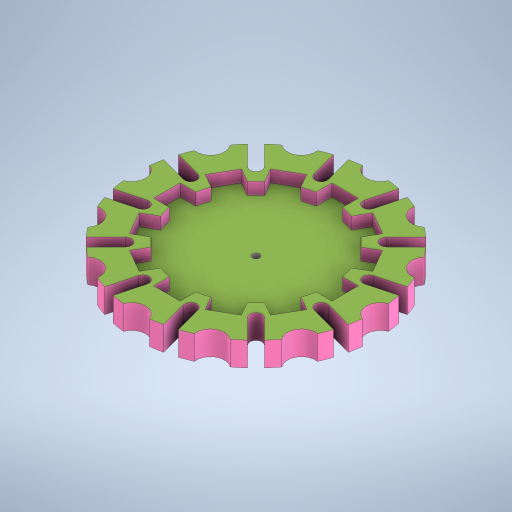
# Autodesk Inventor part: Geneva Gear 12
Saved by Autodesk Inventor 2023 (Build 270158000, 158)
## iProperties
Created: 2022-10-22
Part Number: Geneva Gear 12
Material: Generic
Document SubType Name: Modeling
Designer: annah
Density: 1 g/cm^3
Appearance: Default
Author: annah
Autodesk Inventor part; units mm, degrees
ref_plane "YZ Plane" through (0, 0, 0) normal (1, 0, 0) x (0, 1, 0)
ref_plane "XZ Plane" through (0, 0, 0) normal (0, 1, 0) x (-1, 0, 0)
ref_plane "XY Plane" through (0, 0, 0) normal (0, 0, 1) x (1, 0, 0)
sketch "Sketch1" plane through (0, 0, 0) normal (0, 1, 0) x (-1, 0, 0)
  line L0 (19.1342, -46.194) -> (0, -54.1231)
  line L1 (0, -54.1231) -> (0, 0)
  line L2 (0, 0) -> (19.1342, -46.194)
  circle A0 centre (0, 0) radius 50
  line L3 (17.2491, -28.6141) -> (23.8838, -44.6316)
  circle A1 centre (0, -54.1231) radius 20.712
  arc A2 (17.5355, -29.3054) -> (8.1665, -32.7812) centre (12.7859, -30.8678) ccw
  line L4 (14.5151, -48.1081) -> (8.1665, -32.7812)
  line L5 (19.1342, -41.194) -> (0, -41.194)
  circle A3 centre (0, -54.1231) radius 12.9291
  arc A4 (-11.6961, -48.6128) -> (11.6961, -48.6128) centre (0, 0) ccw
  arc A5 (-11.6961, -48.6128) -> (11.6961, -48.6128) centre (0, -54.1231) ccw
  circle A6 centre (0, -54.1231) radius 32.5
  arc A7 (19.1342, -41.194) -> (16.6765, -41.8397) centre (19.1342, -46.194) ccw
  arc A8 (14.4249, -47.874) -> (23.5974, -43.9403) centre (19.1342, -46.194) ccw
  line L6 (32.4302, -8.0362) -> (48.4477, -14.6709)
  arc A9 (33.1215, -8.3226) -> (28.9544, -17.4053) centre (30.8678, -12.7859) ccw
  line L7 (44.2813, -23.7539) -> (28.9544, -17.4053)
  arc A10 (44.052, -23.6521) -> (47.7564, -14.3846) centre (46.194, -19.1342) ccw
  circle A11 centre (38.2708, -38.2708) radius 12.9291
  line L8 (28.6141, 17.2491) -> (44.6316, 23.8838)
  arc A12 (29.3054, 17.5355) -> (32.7812, 8.1665) centre (30.8678, 12.7859) ccw
  line L9 (48.1081, 14.5151) -> (32.7812, 8.1665)
  arc A13 (47.874, 14.4249) -> (43.9403, 23.5974) centre (46.194, 19.1342) ccw
  circle A14 centre (54.1231, 0) radius 12.9291
  line L10 (8.0362, 32.4302) -> (14.6709, 48.4477)
  arc A15 (8.3226, 33.1215) -> (17.4053, 28.9544) centre (12.7859, 30.8678) ccw
  line L11 (23.7539, 44.2813) -> (17.4053, 28.9544)
  arc A16 (23.6521, 44.052) -> (14.3846, 47.7564) centre (19.1342, 46.194) ccw
  circle A17 centre (38.2708, 38.2708) radius 12.9291
  line L12 (-17.2491, 28.6141) -> (-23.8838, 44.6316)
  arc A18 (-17.5355, 29.3054) -> (-8.1665, 32.7812) centre (-12.7859, 30.8678) ccw
  line L13 (-14.5151, 48.1081) -> (-8.1665, 32.7812)
  arc A19 (-14.4249, 47.874) -> (-23.5974, 43.9403) centre (-19.1342, 46.194) ccw
  circle A20 centre (0, 54.1231) radius 12.9291
  line L14 (-32.4302, 8.0362) -> (-48.4477, 14.6709)
  arc A21 (-33.1215, 8.3226) -> (-28.9544, 17.4053) centre (-30.8678, 12.7859) ccw
  line L15 (-44.2813, 23.7539) -> (-28.9544, 17.4053)
  arc A22 (-44.052, 23.6521) -> (-47.7564, 14.3846) centre (-46.194, 19.1342) ccw
  circle A23 centre (-38.2708, 38.2708) radius 12.9291
  line L16 (-28.6141, -17.2491) -> (-44.6316, -23.8838)
  arc A24 (-29.3054, -17.5355) -> (-32.7812, -8.1665) centre (-30.8678, -12.7859) ccw
  line L17 (-48.1081, -14.5151) -> (-32.7812, -8.1665)
  arc A25 (-47.874, -14.4249) -> (-43.9403, -23.5974) centre (-46.194, -19.1342) ccw
  circle A26 centre (-54.1231, 0) radius 12.9291
  line L18 (-8.0362, -32.4302) -> (-14.6709, -48.4477)
  arc A27 (-8.3226, -33.1215) -> (-17.4053, -28.9544) centre (-12.7859, -30.8678) ccw
  line L19 (-23.7539, -44.2813) -> (-17.4053, -28.9544)
  arc A28 (-23.6521, -44.052) -> (-14.3846, -47.7564) centre (-19.1342, -46.194) ccw
  circle A29 centre (-38.2708, -38.2708) radius 12.9291
  circle A30 centre (0, 0) radius 3.5
  circle A31 centre (0, -54.1231) radius 3.5
  arc A32 (-7.5, -54.1231) -> (7.5, -54.1231) centre (0, -54.1231) ccw
  arc A33 (7.5, 0) -> (-7.5, 0) centre (0, 0) ccw
  line L20 (7.5, 0) -> (7.5, -54.1231)
  line L21 (-7.5, 0) -> (-7.5, -54.1231)
  circle A34 centre (0, -33.4111) radius 5
  point P0 (8.1662, -32.7805)
  point P1 (23.5974, -43.9403)
  point P2 (28.9537, -17.405)
  point P3 (29.1285, -29.1285)
  point P4 (26.1041, -42.6448)
  point P5 (42.6448, -26.1041)
  point P6 (32.7805, 8.1662)
  point P7 (41.194, 0)
  point P8 (48.6128, -11.6961)
  point P9 (48.6128, 11.6961)
  point P10 (17.405, 28.9537)
  point P11 (29.1285, 29.1285)
  point P12 (42.6448, 26.1041)
  point P13 (26.1041, 42.6448)
  point P14 (-8.1662, 32.7805)
  point P15 (0, 41.194)
  point P16 (11.6961, 48.6128)
  point P17 (-11.6961, 48.6128)
  point P18 (-28.9537, 17.405)
  point P19 (-29.1285, 29.1285)
  point P20 (-26.1041, 42.6448)
  point P21 (-42.6448, 26.1041)
  point P22 (-32.7805, -8.1662)
  point P23 (-41.194, 0)
  point P24 (-48.6128, 11.6961)
  point P25 (-48.6128, -11.6961)
  point P26 (-17.405, -28.9537)
  point P27 (-29.1285, -29.1285)
  point P28 (-42.6448, -26.1041)
  point P29 (-26.1041, -42.6448)
  point P30 (23.6521, -44.052)
  point P31 (26.1041, -42.6448)
  point P32 (42.6448, -26.1041)
  point P33 (44.049, -23.6577)
  point P34 (47.874, -14.4249)
  point P35 (48.6128, -11.6961)
  point P36 (48.6128, 11.6961)
  point P37 (47.8758, 14.4189)
  point P38 (44.052, 23.6521)
  point P39 (42.6448, 26.1041)
  point P40 (26.1041, 42.6448)
  point P41 (23.6577, 44.049)
  point P42 (14.4249, 47.874)
  point P43 (11.6961, 48.6128)
  point P44 (-11.6961, 48.6128)
  point P45 (-14.4189, 47.8758)
  point P46 (-23.6521, 44.052)
  point P47 (-26.1041, 42.6448)
  point P48 (-42.6448, 26.1041)
  point P49 (-44.049, 23.6577)
  point P50 (-47.874, 14.4249)
  point P51 (-48.6128, 11.6961)
  point P52 (-48.6128, -11.6961)
  point P53 (-47.8758, -14.4189)
  point P54 (-44.052, -23.6521)
  point P55 (-42.6448, -26.1041)
  point P56 (-26.1041, -42.6448)
  point P57 (-23.6577, -44.049)
  point P58 (-14.4249, -47.874)
  point P59 (14.4189, -47.8758)
  dimension "d2" = 100
  dimension "d3" = 22.5
  dimension "d4" = 20.712
  dimension "d5" = 50
  dimension "d6" = 54.1231
  dimension "d7" = 10
  dimension "d8" = 25.8582
  dimension "d9" = 65
  dimension "d10" = 360
  dimension "d11" = 7
  dimension "d12" = 7
  dimension "d13" = 15
  dimension "d14" = 15
  dimension "d15" = 10
  constraints: 113 point on circle, 44 end point, 35 centre point, 28 point on line, 9 coincident, 3 tangent, 2 vertical, 1 concentric, 1 parallel, 1 perpendicular, 161 other
  measures "d2" diameter of A0
  measures "d3" angle of L2 L1
  measures "d4" distance of L0.start L0.end
  measures "d5" distance of L1.end L0.start
  measures "d6" distance of L0.end L1.end
  measures "d7" diameter of A2
  measures "d8" diameter of A3
  measures "d9" diameter of A6
  measures "d11" diameter of A30
  measures "d12" diameter of A31
  measures "d13" diameter of A32
  measures "d14" diameter of A33
  measures "d15" diameter of A34
sketch "Sketch2" plane through (0, 0, 0) normal (0, 1, 0) x (-1, 0, 0)
  circle A0 centre (0, 0) radius 100
  line L0 (0, 0) -> (18.5658, -69.2885)
  line L1 (0, 0) -> (0, -103.5276)
  arc A1 (24.6448, -72.6673) -> (14.9907, -75.2542) centre (0, 0) ccw
  circle A2 centre (25.8819, -96.5926) radius 5
  arc A3 (24.729, -72.9816) -> (15.0747, -75.5678) centre (19.8599, -74.1181) ccw
  line L2 (30.6777, -95.1782) -> (24.6448, -72.6673)
  line L3 (21.0523, -97.8867) -> (14.9907, -75.2542)
  circle A4 centre (0, -103.5276) radius 11.6229
  line L4 (21.0523, -97.8867) -> (25.8819, -96.5926)
  arc A5 (-25.8819, -96.5926) -> (26.7197, -101.5219) centre (0, -103.5276) ccw
  circle A6 centre (0, -103.5276) radius 40
  arc A7 (57.9067, -50.8394) -> (50.8389, -57.9063) centre (54.2582, -54.2582) ccw
  line L5 (67.1751, -74.2462) -> (50.6094, -57.6767)
  line L6 (74.1567, -67.0879) -> (57.6767, -50.6094)
  circle A8 centre (70.7107, -70.7107) radius 5
  circle A9 centre (51.7638, -89.6575) radius 11.6229
  arc A10 (75.5684, -15.0748) -> (72.9809, -24.7289) centre (74.1181, -19.8599) ccw
  line L7 (95.2985, -30.7115) -> (72.6673, -24.6448)
  line L8 (97.7655, -21.0214) -> (75.2542, -14.9907)
  circle A11 centre (96.5926, -25.8819) radius 5
  circle A12 centre (89.6575, -51.7638) radius 11.6229
  arc A13 (72.9816, 24.729) -> (75.5678, 15.0747) centre (74.1181, 19.8599) ccw
  line L9 (97.8867, 21.0523) -> (75.2542, 14.9907)
  line L10 (95.1782, 30.6777) -> (72.6673, 24.6448)
  circle A14 centre (96.5926, 25.8819) radius 5
  circle A15 centre (103.5276, 0) radius 11.6229
  arc A16 (50.8394, 57.9067) -> (57.9063, 50.8389) centre (54.2582, 54.2582) ccw
  line L11 (74.2462, 67.1751) -> (57.6767, 50.6094)
  line L12 (67.0879, 74.1567) -> (50.6094, 57.6767)
  circle A17 centre (70.7107, 70.7107) radius 5
  circle A18 centre (89.6575, 51.7638) radius 11.6229
  arc A19 (15.0748, 75.5684) -> (24.7289, 72.9809) centre (19.8599, 74.1181) ccw
  line L13 (30.7115, 95.2985) -> (24.6448, 72.6673)
  line L14 (21.0214, 97.7655) -> (14.9907, 75.2542)
  circle A20 centre (25.8819, 96.5926) radius 5
  circle A21 centre (51.7638, 89.6575) radius 11.6229
  arc A22 (-24.729, 72.9816) -> (-15.0747, 75.5678) centre (-19.8599, 74.1181) ccw
  line L15 (-21.0523, 97.8867) -> (-14.9907, 75.2542)
  line L16 (-30.6777, 95.1782) -> (-24.6448, 72.6673)
  circle A23 centre (-25.8819, 96.5926) radius 5
  circle A24 centre (0, 103.5276) radius 11.6229
  arc A25 (-57.9067, 50.8394) -> (-50.8389, 57.9063) centre (-54.2582, 54.2582) ccw
  line L17 (-67.1751, 74.2462) -> (-50.6094, 57.6767)
  line L18 (-74.1567, 67.0879) -> (-57.6767, 50.6094)
  circle A26 centre (-70.7107, 70.7107) radius 5
  circle A27 centre (-51.7638, 89.6575) radius 11.6229
  arc A28 (-75.5684, 15.0748) -> (-72.9809, 24.7289) centre (-74.1181, 19.8599) ccw
  line L19 (-95.2985, 30.7115) -> (-72.6673, 24.6448)
  line L20 (-97.7655, 21.0214) -> (-75.2542, 14.9907)
  circle A29 centre (-96.5926, 25.8819) radius 5
  circle A30 centre (-89.6575, 51.7638) radius 11.6229
  arc A31 (-72.9816, -24.729) -> (-75.5678, -15.0747) centre (-74.1181, -19.8599) ccw
  line L21 (-97.8867, -21.0523) -> (-75.2542, -14.9907)
  line L22 (-95.1782, -30.6777) -> (-72.6673, -24.6448)
  circle A32 centre (-96.5926, -25.8819) radius 5
  circle A33 centre (-103.5276, 0) radius 11.6229
  arc A34 (-50.8394, -57.9067) -> (-57.9063, -50.8389) centre (-54.2582, -54.2582) ccw
  line L23 (-74.2462, -67.1751) -> (-57.6767, -50.6094)
  line L24 (-67.0879, -74.1567) -> (-50.6094, -57.6767)
  circle A35 centre (-70.7107, -70.7107) radius 5
  circle A36 centre (-89.6575, -51.7638) radius 11.6229
  arc A37 (-15.0748, -75.5684) -> (-24.7289, -72.9809) centre (-19.8599, -74.1181) ccw
  line L25 (-30.7115, -95.2985) -> (-24.6448, -72.6673)
  line L26 (-21.0214, -97.7655) -> (-14.9907, -75.2542)
  circle A38 centre (-25.8819, -96.5926) radius 5
  circle A39 centre (-51.7638, -89.6575) radius 11.6229
  circle A40 centre (0, 0) radius 3
  circle A41 centre (0, -103.5276) radius 2.5
  point P0 (50.7227, -50.7227)
  point P1 (73.9009, -74.5607)
  point P2 (69.2885, -18.5658)
  point P3 (101.2804, -27.621)
  point P4 (69.2885, 18.5658)
  point P5 (101.5219, 26.7197)
  point P6 (50.7227, 50.7227)
  point P7 (74.5607, 73.9009)
  point P8 (18.5658, 69.2885)
  point P9 (27.621, 101.2804)
  point P10 (-18.5658, 69.2885)
  point P11 (-26.7197, 101.5219)
  point P12 (-50.7227, 50.7227)
  point P13 (-73.9009, 74.5607)
  point P14 (-69.2885, 18.5658)
  point P15 (-101.2804, 27.621)
  point P16 (-69.2885, -18.5658)
  point P17 (-101.5219, -26.7197)
  point P18 (-50.7227, -50.7227)
  point P19 (-74.5607, -73.9009)
  point P20 (-18.5658, -69.2885)
  point P21 (-27.621, -101.2804)
  point P22 (40.2917, -91.5236)
  point P23 (59.1159, -80.6555)
  point P24 (67.0867, -74.1578)
  point P25 (80.6555, -59.1159)
  point P26 (91.5236, -40.2917)
  point P27 (95.1777, -30.6791)
  point P28 (99.4077, -10.8682)
  point P29 (99.4077, 10.8682)
  point P30 (97.7659, 21.0199)
  point P31 (91.5236, 40.2917)
  point P32 (80.6555, 59.1159)
  point P33 (74.1578, 67.0867)
  point P34 (59.1159, 80.6555)
  point P35 (40.2917, 91.5236)
  point P36 (30.6791, 95.1777)
  point P37 (10.8682, 99.4077)
  point P38 (-10.8682, 99.4077)
  point P39 (-21.0199, 97.7659)
  point P40 (-40.2917, 91.5236)
  point P41 (-59.1159, 80.6555)
  point P42 (-67.0867, 74.1578)
  point P43 (-80.6555, 59.1159)
  point P44 (-91.5236, 40.2917)
  point P45 (-95.1777, 30.6791)
  point P46 (-99.4077, 10.8682)
  point P47 (-99.4077, -10.8682)
  point P48 (-97.7659, -21.0199)
  point P49 (-91.5236, -40.2917)
  point P50 (-80.6555, -59.1159)
  point P51 (-74.1578, -67.0867)
  point P52 (-59.1159, -80.6555)
  point P53 (-40.2917, -91.5236)
  point P54 (-30.6791, -95.1777)
  point P55 (-10.8682, -99.4077)
  point P56 (10.8682, -99.4077)
  point P57 (21.0199, -97.7659)
  dimension "d16" = 200
  dimension "d17" = 15
  dimension "d20" = 10
  dimension "d21" = 10
  dimension "d22" = 80
  dimension "d25" = 360
  dimension "d27" = 6
  dimension "d28" = 5
  constraints: 100 point on circle, 54 end point, 41 centre point, 25 point on line, 8 coincident, 1 vertical, 198 other
  measures "d17" angle of L1 L0
  measures "d20" diameter of A2
  measures "d21" diameter of A3
  measures "d22" diameter of A6
  measures "d27" diameter of A40
  measures "d28" diameter of A41
extrude "Extrusion1" add sketch "Sketch2" along normal blind 20 contours L26 A37 A1 L1 A4 A0 | A0 A6 A1 A37 L25 | A0 A39 L24 A34 A1 A6 | L1 A1 A3 L3 A0 A4 | A37 A6 L1 A1 | A6 A37 A1 | A1 A34 A31 A28 A25 A22 A19 A16 A13 A10 A7 A6 A3 L0 A40 L1 A37 | L1 A6 L0 A3 A1 | A6 A1 A7 L5 A0 A9 | A0 L2 A3 A1 A6 | L1 A40 L0 A6 | A34 L23 A0 A36 L22 A31 A1 | A1 A3 A6 | A6 A3 L0 | A31 L21 A0 A33 L20 A28 A1 | A1 A10 L7 A0 A12 L6 A7 | A28 L19 A0 A30 L18 A25 A1 | A1 A13 L9 A0 A15 L8 A10 | A25 L17 A0 A27 L16 A22 A1 | A1 A16 L11 A0 A18 L10 A13 | A22 L15 A0 A24 L14 A19 A1 | A1 A19 L13 A0 A21 L12 A16 picked at (-24.7526, -72.3861)
sketch "Sketch3" plane through (0, 20, 0) normal (0, 1, 0) x (1, 0, 0)
  circle A0 centre (0, 0) radius 3 projected
  line L0 (-11.0031, 74.0969) -> (11.0031, 74.0969)
  line L1 (11.0031, 74.0969) -> (11.0031, 56.269)
  line L2 (11.0031, 56.269) -> (-11.0031, 56.269)
  line L3 (-11.0031, 56.269) -> (-11.0031, 74.0969)
  line L4 (11.0031, 74.0969) -> (0, 65.183) construction
  line L5 (-27.5195, 69.6713) -> (-18.6056, 54.232)
  line L6 (-18.6056, 54.232) -> (-37.6635, 43.2289)
  line L7 (-37.6635, 43.2289) -> (-46.5774, 58.6682)
  line L8 (-46.5774, 58.6682) -> (-27.5195, 69.6713)
  line L9 (-58.6682, 46.5774) -> (-43.2289, 37.6635)
  line L10 (-43.2289, 37.6635) -> (-54.232, 18.6056)
  line L11 (-54.232, 18.6056) -> (-69.6713, 27.5195)
  line L12 (-69.6713, 27.5195) -> (-58.6682, 46.5774)
  line L13 (-74.0969, 11.0031) -> (-56.269, 11.0031)
  line L14 (-56.269, 11.0031) -> (-56.269, -11.0031)
  line L15 (-56.269, -11.0031) -> (-74.0969, -11.0031)
  line L16 (-74.0969, -11.0031) -> (-74.0969, 11.0031)
  line L17 (-69.6713, -27.5195) -> (-54.232, -18.6056)
  line L18 (-54.232, -18.6056) -> (-43.2289, -37.6635)
  line L19 (-43.2289, -37.6635) -> (-58.6682, -46.5774)
  line L20 (-58.6682, -46.5774) -> (-69.6713, -27.5195)
  line L21 (-46.5774, -58.6682) -> (-37.6635, -43.2289)
  line L22 (-37.6635, -43.2289) -> (-18.6056, -54.232)
  line L23 (-18.6056, -54.232) -> (-27.5195, -69.6713)
  line L24 (-27.5195, -69.6713) -> (-46.5774, -58.6682)
  line L25 (-11.0031, -74.0969) -> (-11.0031, -56.269)
  line L26 (-11.0031, -56.269) -> (11.0031, -56.269)
  line L27 (11.0031, -56.269) -> (11.0031, -74.0969)
  line L28 (11.0031, -74.0969) -> (-11.0031, -74.0969)
  line L29 (27.5195, -69.6713) -> (18.6056, -54.232)
  line L30 (18.6056, -54.232) -> (37.6635, -43.2289)
  line L31 (37.6635, -43.2289) -> (46.5774, -58.6682)
  line L32 (46.5774, -58.6682) -> (27.5195, -69.6713)
  line L33 (58.6682, -46.5774) -> (43.2289, -37.6635)
  line L34 (43.2289, -37.6635) -> (54.232, -18.6056)
  line L35 (54.232, -18.6056) -> (69.6713, -27.5195)
  line L36 (69.6713, -27.5195) -> (58.6682, -46.5774)
  line L37 (74.0969, -11.0031) -> (56.269, -11.0031)
  line L38 (56.269, -11.0031) -> (56.269, 11.0031)
  line L39 (56.269, 11.0031) -> (74.0969, 11.0031)
  line L40 (74.0969, 11.0031) -> (74.0969, -11.0031)
  line L41 (69.6713, 27.5195) -> (54.232, 18.6056)
  line L42 (54.232, 18.6056) -> (43.2289, 37.6635)
  line L43 (43.2289, 37.6635) -> (58.6682, 46.5774)
  line L44 (58.6682, 46.5774) -> (69.6713, 27.5195)
  line L45 (46.5774, 58.6682) -> (37.6635, 43.2289)
  line L46 (37.6635, 43.2289) -> (18.6056, 54.232)
  line L47 (18.6056, 54.232) -> (27.5195, 69.6713)
  line L48 (27.5195, 69.6713) -> (46.5774, 58.6682)
  arc A1 (-11.0031, 60.9667) -> (-20.9544, 58.3003) centre (0, 0) ccw
  arc A2 (20.9544, 58.3003) -> (11.0031, 60.9667) centre (0, 0) ccw
  arc A3 (47.2972, 40.0123) -> (40.0123, 47.2972) centre (0, 0) ccw
  arc A4 (-40.0123, 47.2972) -> (-47.2972, 40.0123) centre (0, 0) ccw
  arc A5 (-58.3003, 20.9544) -> (-60.9667, 11.0031) centre (0, 0) ccw
  arc A6 (-60.9667, -11.0031) -> (-58.3003, -20.9544) centre (0, 0) ccw
  arc A7 (-47.2972, -40.0123) -> (-40.0123, -47.2972) centre (0, 0) ccw
  arc A8 (-20.9544, -58.3003) -> (-11.0031, -60.9667) centre (0, 0) ccw
  arc A9 (11.0031, -60.9667) -> (20.9544, -58.3003) centre (0, 0) ccw
  arc A10 (40.0123, -47.2972) -> (47.2972, -40.0123) centre (0, 0) ccw
  arc A11 (58.3003, -20.9544) -> (60.9667, -11.0031) centre (0, 0) ccw
  arc A12 (60.9667, 11.0031) -> (58.3003, 20.9544) centre (0, 0) ccw
  dimension "d36" = 360
  constraints: 98 end point, 24 point on circle, 24 point on line, 12 centre point, 3 coincident, 2 parallel, 1 horizontal, 1 perpendicular, 97 other
extrude "Extrusion2" cut sketch "Sketch3" against normal blind 10
body "Solid1"
